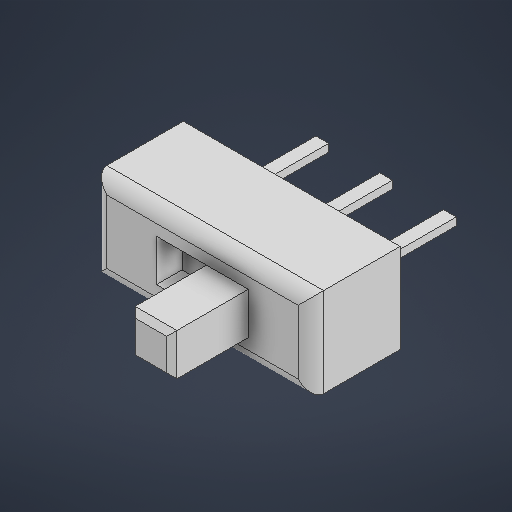
# Autodesk Inventor part: switch
Saved by Autodesk Inventor 2025.2 (Build 292293000, 293)
## iProperties
Created: 2025-12-13
Part Number: switch
Material: Generic
Document SubType Name: Modeling
Designer: sam
Density: 1 g/cm^3
Appearance: Default
Author: sam
Autodesk Inventor part; units mm, degrees
ref_plane "YZ Plane" through (0, 0, 0) normal (1, 0, 0) x (0, 1, 0)
ref_plane "XZ Plane" through (0, 0, 0) normal (0, 1, 0) x (-1, 0, 0)
ref_plane "XY Plane" through (0, 0, 0) normal (0, 0, 1) x (1, 0, 0)
sketch "Sketch1" plane through (0, 0, 0) normal (0, 0, 1) x (1, 0, 0)
  line L0 (4.25, 1.75) -> (-4.25, 1.75)
  line L1 (-4.25, 1.75) -> (-4.25, -1.75)
  line L2 (-4.25, -1.75) -> (4.25, -1.75)
  line L3 (4.25, -1.75) -> (4.25, 1.75)
  line L4 (4.25, 1.75) -> (-4.25, -1.75) construction
  line L5 (-4.25, 1.75) -> (4.25, -1.75) construction
  point P0 (0, 0)
  dimension "d0" = 8.5
  dimension "d1" = 3.5
  constraints: 12 end point, 2 midpoint, 2 parallel, 1 horizontal, 1 perpendicular
  measures "d0" distance of L2.end L1.end
  measures "d1" distance of L1.end L0.end
extrude "Extrusion1" add sketch "Sketch1" along normal blind 3.5
sketch "Sketch2" plane through (0, 0, 3.5) normal (0, 0, 1) x (1, 0, 0)
  line L0 (1.8, 0.82) -> (-1.8, 0.82)
  line L1 (-1.8, 0.82) -> (-1.8, -0.82)
  line L2 (-1.8, -0.82) -> (1.8, -0.82)
  line L3 (1.8, -0.82) -> (1.8, 0.82)
  line L4 (1.8, 0.82) -> (-1.8, -0.82) construction
  line L5 (-1.8, 0.82) -> (1.8, -0.82) construction
  point P0 (0, 0)
  dimension "d4" = 3.6
  dimension "d5" = 1.64
  constraints: 12 end point, 2 midpoint, 2 parallel, 1 horizontal, 1 perpendicular
  measures "d4" distance of L2.end L1.end
  measures "d5" distance of L1.end L0.end
extrude "Extrusion2" cut sketch "Sketch2" against normal blind 1
sketch "Sketch3" plane through (0, 0, 2.5) normal (0, 0, 1) x (1, 0, 0)
  line L0 (-1.8, -0.82) -> (-1.8, 0.82) projected
  line L1 (1.8, -0.82) -> (-1.8, -0.82) projected
  line L2 (1.8, 0.82) -> (1.8, -0.82) projected
  line L3 (-1.8, 0.82) -> (1.8, 0.82) projected
  line L4 (1.8, 0.82) -> (0.16, 0.82)
  line L5 (0.16, 0.82) -> (0.16, -0.82)
  line L6 (0.16, -0.82) -> (1.8, -0.82)
  line L7 (1.8, -0.82) -> (1.8, 0.82)
  point P0 (0, 0)
  dimension "d8" = 1.64
  constraints: 8 end point, 2 parallel, 1 horizontal, 1 perpendicular, 1 point on line
  measures "d8" distance of L6.end L5.end
extrude "Extrusion3" add sketch "Sketch3" along normal blind 4 contours L5 L3 L2 L1
fillet "Fillet1" radius 0.5 4 edges at (0, 1.75, 3.5) (-4.25, 0, 3.5) (0, -1.75, 3.5) (4.25, 0, 3.5)
chamfer "Chamfer1" distance 0.2 angle 45 4 edges at (0.98, 0.82, 6.5) (0.16, 0, 6.5) (0.98, -0.82, 6.5) (1.8, 0, 6.5)
sketch "Sketch4" plane through (0, 0, 0) normal (0, 0, -1) x (-1, 0, 0)
  line L0 (-2.75, 0.15) -> (-2.25, 0.15)
  line L1 (-2.25, 0.15) -> (-2.25, -0.15)
  line L2 (-2.25, -0.15) -> (-2.75, -0.15)
  line L3 (-2.75, -0.15) -> (-2.75, 0.15)
  line L4 (-0.25, 0.15) -> (0.25, 0.15)
  line L5 (0.25, 0.15) -> (0.25, -0.15)
  line L6 (0.25, -0.15) -> (-0.25, -0.15)
  line L7 (-0.25, -0.15) -> (-0.25, 0.15)
  line L8 (2.25, 0.15) -> (2.75, 0.15)
  line L9 (2.75, 0.15) -> (2.75, -0.15)
  line L10 (2.75, -0.15) -> (2.25, -0.15)
  line L11 (2.25, -0.15) -> (2.25, 0.15)
  point P0 (0, 0)
  point P1 (0, 0.15)
  point P2 (-2.5, 0.15)
  point P3 (2.5, 0.15)
  dimension "d15" = 0.5
  dimension "d16" = 0.3
  dimension "d17" = 0.5
  dimension "d18" = 0.3
  dimension "d19" = 0.5
  dimension "d20" = 0.3
  dimension "d21" = 2.5
  dimension "d22" = 2.5
  dimension "d24" = 0.15
  dimension "d25" = 0.25
  constraints: 24 end point, 6 parallel, 3 horizontal, 3 midpoint, 3 perpendicular, 1 point on line
  measures "d15" distance of L1.end L2.end
  measures "d16" distance of L0.end L1.end
  measures "d17" distance of L5.end L6.end
  measures "d18" distance of L4.end L5.end
  measures "d19" distance of L9.end L10.end
  measures "d20" distance of L8.end L9.end
  measures "d21" distance of point (0, 0.15) point (-2.5, 0.15)
  measures "d22" distance of point (2.5, 0.15) point (0, 0.15)
  measures "d24" distance from line of point (0, 0) L4
  measures "d25" distance from line of point (0, 0) L7
extrude "Extrusion4" add sketch "Sketch4" along normal blind 3.7
body "Solid1"
